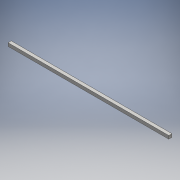
# Autodesk Inventor part: Desk glass holding bar
Saved by Autodesk Inventor 2016 (Build 200138000, 138)
## iProperties
Created: 2015-11-19
Part Number: Desk glass holding bar
Material: 常规
Document SubType Name: Modeling
Designer: Shawn Shi Feng
Density: 1 g/cm^3
Appearance: 默认
Author: Shawn Shi Feng
Autodesk Inventor part; units mm, degrees
ref_plane "YZ Plane" through (0, 0, 0) normal (1, 0, 0) x (0, 1, 0)
ref_plane "XZ Plane" through (0, 0, 0) normal (0, 1, 0) x (-1, 0, 0)
ref_plane "XY Plane" through (0, 0, 0) normal (0, 0, 1) x (1, 0, 0)
sketch "草图1" plane through (0, 0, 0) normal (0, 0, 1) x (1, 0, 0)
  line L0 (-375.051, 60.526) -> (379.949, 60.526)
  line L1 (379.949, 60.526) -> (379.949, 45.526)
  line L2 (379.949, 45.526) -> (-375.051, 45.526)
  line L3 (-375.051, 45.526) -> (-375.051, 60.526)
  point P0 (0, 0)
  dimension "d0" = 755
  dimension "d1" = 15
  constraints: 8 end point, 2 parallel, 1 horizontal, 1 perpendicular
  measures "d0" distance of L0.start L0.end
  measures "d1" distance of L0.end L1.end
extrude "拉伸1" add sketch "草图1" along normal blind 15
sketch "草图2" plane through (379.949, 45.526, 0) normal (1, 0, 0) x (0, 0, -1)
  line L0 (0, 0) -> (0, 15) projected
  line L1 (0, 15) -> (-15, 15) projected
  circle A0 centre (-7.5, 7.5) radius 2.5
  point P0 (0, -45.526)
  dimension "d4" = 7.5
  dimension "d5" = 7.5
  dimension "d6" = 5
  constraints: 1 centre point, 1 coincident
  measures "d4" distance from line of L0 point (-7.5, 7.5)
  measures "d5" distance from line of L1 point (-7.5, 7.5)
  measures "d6" diameter of A0
extrude "拉伸2" cut sketch "草图2" against normal blind 800
